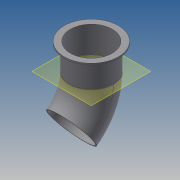
# Autodesk Inventor part: P013_Canon_venturiCoudé
Saved by Autodesk Inventor 2021.3 (Build 253353000, 353)
## iProperties
Created: 2021-10-22
Part Number: P013_Canon_venturiCoudé
Material: Générique
Document SubType Name: Modeling
Designer: gabri
Density: 1 g/cm^3
Appearance: Par défaut
Author: gabri
Autodesk Inventor part; units mm, degrees
ref_plane "YZ Plane" through (0, 0, 0) normal (1, 0, 0) x (0, 1, 0)
ref_plane "XZ Plane" through (0, 0, 0) normal (0, 1, 0) x (-1, 0, 0)
ref_plane "XY Plane" through (0, 0, 0) normal (0, 0, 1) x (1, 0, 0)
sketch "Esquisse2" plane through (0, 0, 0) normal (0, 0, 1) x (1, 0, 0)
  circle A0 centre (0, 0) radius 16
  circle A1 centre (0, 0) radius 13
  dimension "d0" = 32
  dimension "d1" = 26
  constraints: 2 centre point, 2 coincident
  measures "d0" diameter of A0
  measures "d1" diameter of A1
extrude "Extrusion1" add sketch "Esquisse2" along normal blind 1
sketch "Esquisse3" plane through (0, 0, 1) normal (0, 0, 1) x (1, 0, 0)
  circle A0 centre (0, 0) radius 12.4
  circle A1 centre (0, 0) radius 13
  dimension "d6" = 26
  dimension "d7" = 24.8
  constraints: 2 centre point, 2 coincident
  measures "d6" diameter of A1
  measures "d7" diameter of A0
extrude "Extrusion2" add sketch "Esquisse3" against normal blind 15.8
sketch "Esquisse4" plane through (0, 0, 0) normal (1, 0, 0) x (0, 1, 0)
  line L0 (12.4, -14.8) -> (-12.4, -14.8) construction
  line L1 (-12.4, 1) -> (12.4, 1) construction
  arc A0 (-12, -37.8) -> (0, -14.8) centre (-28.0417, -14.8) ccw
  line L2 (0, -67.4158) -> (0, 12.4026) construction
  line L3 (0, -14.8) -> (0, -44.8) construction
  line L4 (22.3657, -42.8417) -> (-48.6343, -42.8417) construction
  point P0 (0, 0)
  dimension "d9" = 30
  dimension "d10" = 23
  dimension "d17" = 12
  constraints: 4 end point, 2 point on circle, 2 tangent, 1 centre point, 1 horizontal, 1 midpoint, 1 point on line
  measures "d9" distance of L3.start L3.end
  measures "d10" distance from line of A0.start L0
  measures "d17" distance from line of L2 A0.start
ref_plane "Plan de construction1" through (0, 0, -14.5) normal (0, 0, 1) x (1, 0, 0)
sketch "Esquisse6" plane through (0, 0, -14.5) normal (0, 0, 1) x (1, 0, 0)
  circle A0 centre (0, 0) radius 12.4 construction
  circle A1 centre (0, 0) radius 16 construction
  circle A2 centre (0, 0) radius 13 construction
  circle A3 centre (0, 0) radius 12.4
  circle A4 centre (0, 0) radius 13
  dimension "d16" = 24.8
  constraints: 2 centre point, 2 coincident, 2 concentric
  measures "d16" diameter of A0
sweep "Balayage1" add profiles "Esquisse6" path "Esquisse4" separate body
